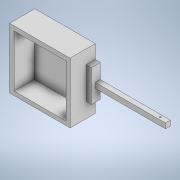
# Autodesk Inventor part: pusher
Saved by Autodesk Inventor 2021 (Build 250183000, 183)
## iProperties
Created: 2021-07-09
Part Number: pusher
Material: Generic
Document SubType Name: Modeling
Designer: Rajeev
Density: 1 g/cm^3
Appearance: Default
Author: Rajeev
Autodesk Inventor part; units mm, degrees
ref_plane "YZ Plane" through (0, 0, 0) normal (1, 0, 0) x (0, 1, 0)
ref_plane "XZ Plane" through (0, 0, 0) normal (0, 1, 0) x (-1, 0, 0)
ref_plane "XY Plane" through (0, 0, 0) normal (0, 0, 1) x (1, 0, 0)
sketch "Sketch5" plane through (0, 0, 0) normal (0, 0, 1) x (1, 0, 0)
  line L0 (-11.1597, 4.6835) -> (8.8403, 4.6835)
  line L1 (8.8403, 4.6835) -> (8.8403, -15.3165)
  line L2 (8.8403, -15.3165) -> (-11.1597, -15.3165)
  line L3 (-11.1597, -15.3165) -> (-11.1597, 4.6835)
  point P0 (0, 0)
  dimension "d13" = 20
  dimension "d14" = 20
  constraints: 8 end point, 2 parallel, 1 horizontal, 1 perpendicular
  measures "d13" distance of L1.end L2.end
  measures "d14" distance of L0.end L1.end
extrude "Extrusion5" add sketch "Sketch5" along normal blind 8
sketch "Sketch6" plane through (0, 0, 8) normal (0, 0, 1) x (1, 0, 0)
  line L0 (-10.6667, 4.1905) -> (8.3333, 4.1905)
  line L1 (8.3333, 4.1905) -> (8.3333, -14.8095)
  line L2 (8.3333, -14.8095) -> (-10.6667, -14.8095)
  line L3 (-10.6667, -14.8095) -> (-10.6667, 4.1905)
  point P0 (0, 0)
  dimension "d17" = 19
  dimension "d18" = 19
  constraints: 8 end point, 2 parallel, 1 horizontal, 1 perpendicular
  measures "d17" distance of L1.end L2.end
  measures "d18" distance of L0.end L1.end
extrude "Extrusion6" cut sketch "Sketch6" against normal blind 7
sketch "Sketch11" plane through (8.8403, -15.3165, 0) normal (1, 0, 0) x (0, 0, -1)
  line L0 (-4.9297, 9.3778) -> (-2.9693, 9.3778)
  line L1 (-2.9693, 9.3778) -> (-2.9693, 11.3958)
  line L2 (-2.9693, 11.3958) -> (-4.9297, 11.3958)
  line L3 (-4.9297, 11.3958) -> (-4.9297, 9.3778)
  point P0 (0, 15.3165)
  constraints: 8 end point, 2 parallel, 1 horizontal, 1 perpendicular
extrude "Extrusion11" add sketch "Sketch11" along normal blind 30
sketch "Sketch12" plane through (8.8403, -5.9387, 2.9693) normal (0, -1, 0) x (1, 0, 0)
  circle A0 centre (26.9647, 0.9802) radius 0.3
  point P0 (-8.8403, -2.9693)
  dimension "d35" = 0.6
  constraints: 1 centre point
  measures "d35" diameter of A0
extrude "Extrusion12" cut sketch "Sketch12" against normal blind 30
sketch "Sketch13" plane through (0, 0, 0) normal (0, 0, -1) x (-1, 0, 0)
  line L0 (-9, 6.898) -> (15, 6.898)
  line L1 (15, 6.898) -> (15, -17.102)
  line L2 (15, -17.102) -> (-9, -17.102)
  line L3 (-9, -17.102) -> (-9, 6.898)
  point P0 (0, 0)
  dimension "d38" = 24
  dimension "d39" = 24
  constraints: 8 end point, 2 parallel, 1 horizontal, 1 perpendicular
  measures "d38" distance of L0.start L0.end
  measures "d39" distance of L0.end L1.end
extrude "Extrusion13" cut sketch "Sketch13" against normal blind 10
sketch "Sketch14" plane through (9, -5.9387, 4.9297) normal (-1, 0, 0) x (0, 0, 1)
  line L0 (-1.9603, 0) -> (-1.9603, 2.018) projected
  line L1 (-1.9603, -10.5808) -> (8.0397, -10.5808)
  line L2 (8.0397, -10.5808) -> (8.0397, 13.4192)
  line L3 (8.0397, 13.4192) -> (-1.9603, 13.4192)
  line L4 (-1.9603, 13.4192) -> (-1.9603, -10.5808)
  point P0 (-4.9297, 5.9387)
  dimension "d42" = 10
  dimension "d43" = 24
  constraints: 8 end point, 2 parallel, 1 horizontal, 1 perpendicular, 1 point on line
  measures "d42" distance of L2.end L3.end
  measures "d43" distance of L3.end L1.start
extrude "Extrusion14" add sketch "Sketch14" along normal blind 24
sketch "Sketch15" plane through (9, -16.5195, 12.9693) normal (0, 0, 1) x (1, 0, 0)
  line L0 (-1.5875, 22.225) -> (-22.225, 22.225)
  line L1 (-22.225, 22.225) -> (-22.225, 1.5875)
  line L2 (-22.225, 1.5875) -> (-1.5875, 1.5875)
  line L3 (-1.5875, 1.5875) -> (-1.5875, 22.225)
  point P0 (-9, 16.5195)
  constraints: 8 end point, 2 parallel, 1 horizontal, 1 perpendicular
extrude "Extrusion15" cut sketch "Sketch15" against normal blind 8
sketch "Sketch16" plane through (9, -5.9387, 4.9297) normal (1, 0, 0) x (0, 0, -1)
  line L0 (1.9603, 13.4192) -> (1.9603, -10.5808) projected
  line L1 (1.9603, 7.9375) -> (-1.5875, 7.9375)
  line L2 (-1.5875, 7.9375) -> (-1.5875, -4.7625)
  line L3 (-1.5875, -4.7625) -> (1.9603, -4.7625)
  line L4 (1.9603, -4.7625) -> (1.9603, 7.9375)
  point P0 (4.9297, 5.9387)
  point P1 (1.9603, -4.7625)
  constraints: 8 end point, 2 parallel, 1 horizontal, 1 perpendicular, 1 point on line
extrude "Extrusion16" add sketch "Sketch16" along normal blind 2
body "Solid2"
